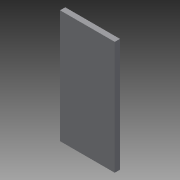
# Autodesk Inventor part: step down
Saved by Autodesk Inventor 2015 (Build 190159000, 159)
## iProperties
Created: 2015-05-05
Part Number: step down
Material: Ogólny
Document SubType Name: Modeling
Designer: Kuba
Density: 1 g/cm^3
Appearance: Domyślna
Author: Kuba
Autodesk Inventor part; units mm, degrees
ref_plane "YZ Plane" through (0, 0, 0) normal (1, 0, 0) x (0, 1, 0)
ref_plane "XZ Plane" through (0, 0, 0) normal (0, 1, 0) x (-1, 0, 0)
ref_plane "XY Plane" through (0, 0, 0) normal (0, 0, 1) x (1, 0, 0)
sketch "Szkic1" plane through (0, 0, 0) normal (0, 1, 0) x (-1, 0, 0)
  line L0 (-10.5, -21.75) -> (10.5, -21.75)
  line L1 (10.5, -21.75) -> (10.5, 21.75)
  line L2 (10.5, 21.75) -> (-10.5, 21.75)
  line L3 (-10.5, 21.75) -> (-10.5, -21.75)
  line L4 (-10.5, -21.75) -> (10.5, 21.75) construction
  line L5 (10.5, -21.75) -> (-10.5, 21.75) construction
  point P0 (0, 0)
  dimension "d0" = 21
  dimension "d1" = 43.5
  constraints: 12 end point, 2 midpoint, 2 parallel, 1 horizontal, 1 perpendicular
  measures "d0" distance of L2.end L1.end
  measures "d1" distance of L1.end L0.end
extrude "Wyciągnięcie proste1" add sketch "Szkic1" along normal blind 2
sketch "Szkic2" plane through (0, 2, 0) normal (0, 1, 0) x (1, 0, 0)
  line L0 (-10.5, 21.75) -> (-10.5, -21.75) projected
  line L1 (-10.5, -21.75) -> (10.5, -21.75) projected
  line L2 (10.5, 21.75) -> (-10.5, 21.75) projected
  line L3 (10.5, -21.75) -> (10.5, 21.75) projected
  point P0 (0, 0)
  point P1 (-7.5, -14.75)
  point P2 (7.5, 15.75)
  dimension "d4" = 3
  dimension "d5" = 7
  dimension "d6" = 6
  dimension "d7" = 3
  measures "d4" distance from line of L0 point (-7.5, -14.75)
  measures "d5" distance from line of L1 point (-7.5, -14.75)
  measures "d6" distance from line of L2 point (7.5, 15.75)
  measures "d7" distance from line of L3 point (7.5, 15.75)
hole "Otwór1" at (-7.5, 2, 14.75) at (7.5, 2, -15.75) direction (0, -1, 0) diameter 3.5 end through all
sketch "Szkic3" plane through (0, 2, 0) normal (0, 1, 0) x (1, 0, 0)
  line L0 (8.25, 11.5) -> (-8.25, 11.5)
  line L1 (-8.25, 11.5) -> (-8.25, -11.5)
  line L2 (-8.25, -11.5) -> (8.25, -11.5)
  line L3 (8.25, -11.5) -> (8.25, 11.5)
  line L4 (8.25, 11.5) -> (-8.25, -11.5) construction
  line L5 (-8.25, 11.5) -> (8.25, -11.5) construction
  point P0 (0, 0)
  dimension "d15" = 16.5
  dimension "d16" = 23
  constraints: 12 end point, 2 midpoint, 2 parallel, 1 horizontal, 1 perpendicular
  measures "d15" distance of L2.end L1.end
  measures "d16" distance of L0.end L1.end
extrude "Wyciągnięcie proste2" add sketch "Szkic3" along normal blind 1.5
sketch "Szkic4" plane through (0, 3.5, 0) normal (0, 1, 0) x (1, 0, 0)
  line L0 (8.25, 11.5) -> (-8.25, 11.5) projected
  line L1 (-8.25, 11.5) -> (-8.25, -11.5) projected
  line L2 (-8.25, -11.5) -> (8.25, -11.5) projected
  line L3 (8.25, -11.5) -> (8.25, 11.5) projected
  circle A0 centre (-5.375, -9.1) radius 0.5
  circle A1 centre (5.375, -9.1) radius 0.5
  circle A2 centre (5.375, 9.1) radius 0.5
  circle A3 centre (-5.375, 9.1) radius 0.5
  circle A4 centre (-4.6129, -1.6011) radius 1.6664
  line L4 (-0.1119, 4.829) -> (-3.4753, 4.829)
  line L5 (-3.4753, 4.829) -> (-3.4753, 3.9387)
  line L6 (-3.4753, 3.9387) -> (-0.1119, 3.9387)
  line L7 (-0.1119, 3.9387) -> (-0.1119, 4.829)
  line L8 (-0.1119, 4.829) -> (-3.4753, 3.9387) construction
  line L9 (-3.4753, 4.829) -> (-0.1119, 3.9387) construction
  point P0 (0, 0)
  point P1 (-1.7936, 4.3838)
  dimension "d19" = 10.75
  dimension "d20" = 10.75
  dimension "d21" = 2.875
  dimension "d22" = 2.875
  dimension "d23" = 2.875
  dimension "d24" = 2.875
  dimension "d25" = 18.2
  dimension "d26" = 18.2
  dimension "d27" = 2.4
  dimension "d28" = 2.4
  dimension "d29" = 2.4
  dimension "d30" = 1
  dimension "d31" = 1
  dimension "d32" = 1
  dimension "d33" = 1
  constraints: 12 end point, 5 centre point, 4 coincident, 2 midpoint, 2 parallel, 1 horizontal, 1 perpendicular
  measures "d19" distance of point (5.375, -9.1) point (-5.375, -9.1)
  measures "d20" distance of point (5.375, 9.1) point (-5.375, 9.1)
  measures "d21" distance from line of L1 point (-5.375, -9.1)
  measures "d22" distance from line of L3 point (5.375, -9.1)
  measures "d23" distance from line of L1 point (-5.375, 9.1)
  measures "d24" distance from line of L3 point (5.375, 9.1)
  measures "d25" distance of point (-5.375, 9.1) point (-5.375, -9.1)
  measures "d26" distance of point (5.375, 9.1) point (5.375, -9.1)
  measures "d27" distance from line of L2 point (-5.375, -9.1)
  measures "d28" distance from line of L0 point (-5.375, 9.1)
  measures "d29" distance from line of L2 point (5.375, -9.1)
  measures "d30" diameter of A0
  measures "d31" diameter of A1
  measures "d32" diameter of A2
  measures "d33" diameter of A3
extrude "Wyciągnięcie proste3" add sketch "Szkic4" along normal blind 3 contours A0 | A1 | A2 | A3 | A4 | L7 L6 L5 L4
sketch "Szkic5" plane through (0, 3.5, 0) normal (0, 1, 0) x (1, 0, 0)
  line L0 (-0.1119, 4.829) -> (-0.1119, 3.9387) projected
  line L1 (-0.1119, 3.9387) -> (-3.4753, 3.9387) projected
  line L2 (-3.4753, 3.9387) -> (-3.4753, 4.829) projected
  line L3 (-3.4753, 4.829) -> (-0.1119, 4.829) projected
  circle A0 centre (5.375, 9.1) radius 0.5 projected
  circle A1 centre (-5.375, -9.1) radius 0.5 projected
  circle A2 centre (5.375, -9.1) radius 0.5 projected
  circle A3 centre (-5.375, 9.1) radius 0.5 projected
  circle A4 centre (-4.6129, -1.6011) radius 1.6664 projected
  line L4 (8.25, 11.5) -> (-8.25, 11.5) projected
  line L5 (-8.25, 11.5) -> (-8.25, -11.5) projected
  line L6 (-8.25, -11.5) -> (8.25, -11.5) projected
  line L7 (8.25, -11.5) -> (8.25, 11.5) projected
  line L8 (7.9153, 5.177) -> (4.875, 5.177)
  line L9 (4.875, 5.177) -> (4.875, -5.177)
  line L10 (4.875, -5.177) -> (7.9153, -5.177)
  line L11 (7.9153, -5.177) -> (7.9153, 5.177)
  line L12 (7.9153, 5.177) -> (4.875, -5.177) construction
  line L13 (4.875, 5.177) -> (7.9153, -5.177) construction
  point P0 (0, 0)
  point P1 (6.3951, 0)
  constraints: 12 end point, 2 midpoint, 2 parallel, 1 horizontal, 1 perpendicular
extrude "Wyciągnięcie proste4" add sketch "Szkic5" along normal blind 10 contours L11 L10 L9 L8
sketch "Szkic6" plane through (0, 2, 0) normal (0, 1, 0) x (1, 0, 0)
  line L0 (7.9153, 5.177) -> (7.9153, -5.177) projected
  line L1 (7.9153, -5.177) -> (4.875, -5.177) projected
  line L2 (4.875, -5.177) -> (4.875, 5.177) projected
  line L3 (4.875, 5.177) -> (7.9153, 5.177) projected
  line L4 (-0.1119, 4.829) -> (-0.1119, 3.9387) projected
  line L5 (-0.1119, 3.9387) -> (-3.4753, 3.9387) projected
  line L6 (-3.4753, 3.9387) -> (-3.4753, 4.829) projected
  line L7 (-3.4753, 4.829) -> (-0.1119, 4.829) projected
  circle A0 centre (5.375, 9.1) radius 0.5 projected
  circle A1 centre (-5.375, -9.1) radius 0.5 projected
  circle A2 centre (5.375, -9.1) radius 0.5 projected
  circle A3 centre (-5.375, 9.1) radius 0.5 projected
  circle A4 centre (-4.6129, -1.6011) radius 1.6664 projected
  line L8 (8.25, 11.5) -> (-8.25, 11.5) projected
  line L9 (-8.25, 11.5) -> (-8.25, -11.5) projected
  line L10 (-8.25, -11.5) -> (8.25, -11.5) projected
  line L11 (8.25, -11.5) -> (8.25, 11.5) projected
  line L12 (8.2581, -13.982) -> (-3.4753, -13.982)
  line L13 (-3.4753, -13.982) -> (-3.4753, -20.203)
  line L14 (-3.4753, -20.203) -> (8.2581, -20.203)
  line L15 (8.2581, -20.203) -> (8.2581, -13.982)
  line L16 (8.2581, -13.982) -> (-3.4753, -20.203) construction
  line L17 (-3.4753, -13.982) -> (8.2581, -20.203) construction
  line L18 (3.4087, 20.8092) -> (-9.3017, 20.8092)
  line L19 (-9.3017, 20.8092) -> (-9.3017, 14.8186)
  line L20 (-9.3017, 14.8186) -> (3.4087, 14.8186)
  line L21 (3.4087, 14.8186) -> (3.4087, 20.8092)
  line L22 (3.4087, 20.8092) -> (-9.3017, 14.8186) construction
  line L23 (-9.3017, 20.8092) -> (3.4087, 14.8186) construction
  point P0 (0, 0)
  point P1 (2.3914, -17.0925)
  point P2 (-2.9465, 17.8139)
  constraints: 24 end point, 4 midpoint, 4 parallel, 2 horizontal, 2 perpendicular
extrude "Wyciągnięcie proste5" add sketch "Szkic6" along normal blind 10 contours L15 L14 L13 L12 | L21 L20 L19 L18
equation "\"d20\" = d19"
equation "\"d21\" = d22"
equation "\"d23\" = d24"
equation "\"d26\" = d25"
equation "\"d27\" = d28"
equation "\"d29\" = d27"
